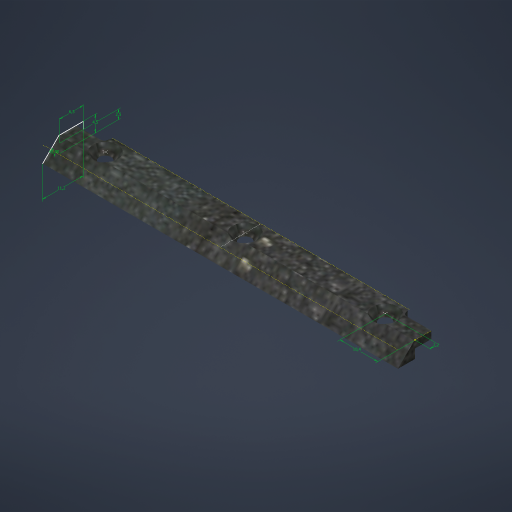
# Autodesk Inventor part: Plog2
Saved by Autodesk Inventor 2023 (Build 270158000, 158)
## iProperties
Created: 2022-01-27
Part Number: Plog2
Material: Stal
Document SubType Name: Modeling
Designer: Michał
Density: 7.85 g/cm^3
Appearance: Płyta
Author: Michał
Autodesk Inventor part; units mm, degrees
ref_plane "YZ Plane" through (0, 0, 0) normal (1, 0, 0) x (0, 1, 0)
ref_plane "XZ Plane" through (0, 0, 0) normal (0, 1, 0) x (-1, 0, 0)
ref_plane "XY Plane" through (0, 0, 0) normal (0, 0, 1) x (1, 0, 0)
sketch "Szkic1" plane through (0, 0, 0) normal (1, 0, 0) x (0, 1, 0)
  line L0 (0, 0) -> (4.5, -4.5)
  line L1 (4.5, -4.5) -> (4.5, -11.2)
  line L2 (4.5, -11.2) -> (2.5, -11.2)
  line L3 (2.5, -11.2) -> (2.5, -4.7)
  line L4 (2.5, -4.7) -> (0, -4.7)
  line L5 (0, -4.7) -> (0, 0)
  line L6 (2.5, -4.7) -> (2.5, -2.5) construction
  dimension "d0" = 11.2
  dimension "d1" = 4.5
  dimension "d2" = 45
  dimension "d3" = 2.5
  dimension "d4" = 6.5
  constraints: 14 end point, 4 perpendicular, 2 vertical, 1 point on line
  measures "d0" distance from line of L2 L0.start
  measures "d1" distance between parallel lines of L5 L1
  measures "d2" angle of L5 L0
  measures "d3" distance of L3.end L4.end
  measures "d4" distance of L2.end L3.end
extrude "Wyciągnięcie proste1" add sketch "Szkic1" along normal blind 98
sketch "Szkic2" plane through (0, 4.5, -4.5) normal (0, 1, 0) x (1, 0, 0)
  line L0 (0, 6.7) -> (0, 0.2) projected
  line L1 (0, 6.7) -> (7.9, 6.7)
  line L2 (7.9, 6.7) -> (7.9, 4.7)
  line L3 (7.9, 4.7) -> (0, 4.7)
  line L4 (0, 4.7) -> (0, 6.7)
  line L5 (0, 0.2) -> (98, 0.2) construction
  line L6 (49, 0.2) -> (49, 6.7) construction
  line L7 (0, 6.7) -> (98, 6.7) construction
  line L8 (98, 6.7) -> (90.1, 6.7)
  line L9 (90.1, 6.7) -> (90.1, 4.7)
  line L10 (90.1, 4.7) -> (98, 4.7)
  line L11 (98, 4.7) -> (98, 6.7)
  point P0 (0, -4.5)
  dimension "d7" = 7.9
  dimension "d8" = 2
  constraints: 18 end point, 3 symmetric about line, 2 midpoint, 2 parallel, 1 horizontal, 1 perpendicular
  measures "d7" distance of L0.start L1.end
  measures "d8" distance between parallel lines of L1 L3
extrude "Wyciągnięcie proste2" cut sketch "Szkic2" against normal through all
sketch "Szkic3" plane through (0, 4.5, -4.5) normal (0, 1, 0) x (1, 0, 0)
  line L0 (0, -4.5) -> (98, -4.5) construction
  line L1 (49, -4.5) -> (49, 6.7) construction
  line L2 (7.9, 6.7) -> (90.1, 6.7) construction
  line L3 (98, 4.7) -> (98, 0) construction
  point P0 (87.6, 2.4)
  point P1 (49, 2.4)
  point P2 (10.4, 2.4)
  point P3 (98, 0.2)
  dimension "d11" = 10.4
  dimension "d21" = 2.2
  constraints: 2 end point, 2 midpoint, 1 horizontal alignment, 1 point on line, 1 symmetric about line
  measures "d11" distance from line of L3 point (87.6, 2.4)
  measures "d21" vertical distance of point (98, 0.2) point (87.6, 2.4)
hole "Otwór1" at (87.6, 4.5, -6.9) at (49, 4.5, -6.9) at (10.4, 4.5, -6.9) direction (0, -1, 0) diameter 3.2 end through all countersink diameter 6.9 countersink angle 84.225 clearance for "Śruba ze łbem stożkowym ISO 2009/7046" size "M3" standard "ISO"
fillet "Zaokrąglenie1" radius 1 4 edges at (90.1, 3.4707, -9.2) (90.1, 3.5, -11.2) (7.9, 3.4707, -9.2) (7.9, 3.5, -11.2)
